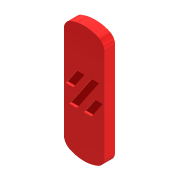
# Autodesk Inventor part: Cover_Squared
Saved by Autodesk Inventor 2021 (Build 250183000, 183)
## iProperties
Created: 2021-09-01
Part Number: Cover_Squared
Material: Generisch
Document SubType Name: Modeling
Designer: Rama
Density: 1 g/cm^3
Appearance: Hellrot
Author: Rama
Autodesk Inventor part; units mm, degrees
ref_plane "YZ Plane" through (0, 0, 0) normal (1, 0, 0) x (0, 1, 0)
ref_plane "XZ Plane" through (0, 0, 0) normal (0, 1, 0) x (-1, 0, 0)
ref_plane "XY Plane" through (0, 0, 0) normal (0, 0, 1) x (1, 0, 0)
sketch "Skizze1" plane through (0, 0, 0) normal (0, 0, 1) x (1, 0, 0)
  line L0 (7.75, -17.6806) -> (7.75, 17.6806) projected
  line L1 (-7.75, 17.6806) -> (-7.75, -17.6806) projected
  circle A0 centre (0, 0) radius 3.025 projected
  arc A1 (-5.3363, -21.3526) -> (5.3363, -21.3526) centre (0, -9) ccw projected
  arc A2 (5.3363, -21.3526) -> (7.75, -17.6806) centre (3.75, -17.6806) ccw projected
  arc A3 (7.75, 17.6806) -> (5.3363, 21.3526) centre (3.75, 17.6806) ccw projected
  arc A4 (5.3363, 21.3526) -> (-5.3363, 21.3526) centre (0, 9) ccw projected
  arc A5 (-5.3363, 21.3526) -> (-7.75, 17.6806) centre (-3.75, 17.6806) ccw projected
  arc A6 (-7.75, -17.6806) -> (-5.3363, -21.3526) centre (-3.75, -17.6806) ccw projected
  circle A7 centre (-0.25, 17) radius 1.7 projected
  circle A8 centre (-0.25, -7) radius 1.7 projected
  line L2 (5.34, 14.1) -> (3.3, 14.1) projected
  line L3 (3.3, 14.1) -> (3.3, 17.74) projected
  line L4 (3.3, 17.74) -> (5.34, 17.74) projected
  line L5 (5.34, 17.74) -> (5.34, 14.1) projected
  line L6 (-3.8, 14.1) -> (-5.84, 14.1) projected
  line L7 (-5.84, 14.1) -> (-5.84, 17.74) projected
  line L8 (-5.84, 17.74) -> (-3.8, 17.74) projected
  line L9 (-3.8, 17.74) -> (-3.8, 14.1) projected
  circle A9 centre (-0.25, -15.278) radius 2.9 projected
  point P0 (0, 0)
  point P1 (-17.1225, -5.975)
  point P2 (-17.1225, -12.025)
  point P3 (-17.1225, 6.3)
  point P4 (-17.1225, -14.3)
  point P5 (-17.1225, -17.7)
  constraints: 1 other
extrude "Extrusion1" add sketch "Skizze1" along normal blind 4 contours A2 A1 A6 L1 A5 A4 A3 L0 | A0 | A7 | A8 | L2 L3 L4 L5 | L6 L7 L8 L9 | A9
sketch "Skizze2" plane through (0, 0, 0) normal (0, 0, -1) x (-1, 0, 0)
  circle A0 centre (0, 0) radius 3.025 projected
  arc A1 (-5.3363, -21.3526) -> (5.3363, -21.3526) centre (0, -9) ccw projected
  arc A2 (-7.75, -17.6806) -> (-5.3363, -21.3526) centre (-3.75, -17.6806) ccw projected
  line L0 (-7.75, -17.6806) -> (-7.75, 17.6806) projected
  arc A3 (-5.3363, 21.3526) -> (-7.75, 17.6806) centre (-3.75, 17.6806) ccw projected
  arc A4 (5.3363, 21.3526) -> (-5.3363, 21.3526) centre (0, 9) ccw projected
  arc A5 (7.75, 17.6806) -> (5.3363, 21.3526) centre (3.75, 17.6806) ccw projected
  line L1 (7.75, 17.6806) -> (7.75, -17.6806) projected
  arc A6 (5.3363, -21.3526) -> (7.75, -17.6806) centre (3.75, -17.6806) ccw projected
  circle A7 centre (0.25, 17) radius 1.7 projected
  circle A8 centre (0.25, -7) radius 1.7 projected
  line L2 (-5.34, 14.1) -> (-3.3, 14.1) projected
  line L3 (-3.3, 14.1) -> (-3.3, 17.74) projected
  line L4 (-3.3, 17.74) -> (-5.34, 17.74) projected
  line L5 (-5.34, 17.74) -> (-5.34, 14.1) projected
  line L6 (3.8, 14.1) -> (5.84, 14.1) projected
  line L7 (5.84, 14.1) -> (5.84, 17.74) projected
  line L8 (5.84, 17.74) -> (3.8, 17.74) projected
  line L9 (3.8, 17.74) -> (3.8, 14.1) projected
  circle A9 centre (0.25, -15.278) radius 2.9 projected
  point P0 (0, 0)
extrude "Extrusion2" cut sketch "Skizze2" against normal blind 3.1 contours A0
sketch "Skizze3" plane through (0, 0, 0) normal (0, 0, -1) x (-1, 0, 0)
  circle A0 centre (0, 0) radius 3.025 projected
  arc A1 (-5.3363, -21.3526) -> (5.3363, -21.3526) centre (0, -9) ccw projected
  arc A2 (-7.75, -17.6806) -> (-5.3363, -21.3526) centre (-3.75, -17.6806) ccw projected
  line L0 (-7.75, -17.6806) -> (-7.75, 17.6806) projected
  arc A3 (-5.3363, 21.3526) -> (-7.75, 17.6806) centre (-3.75, 17.6806) ccw projected
  arc A4 (5.3363, 21.3526) -> (-5.3363, 21.3526) centre (0, 9) ccw projected
  arc A5 (7.75, 17.6806) -> (5.3363, 21.3526) centre (3.75, 17.6806) ccw projected
  line L1 (7.75, 17.6806) -> (7.75, -17.6806) projected
  arc A6 (5.3363, -21.3526) -> (7.75, -17.6806) centre (3.75, -17.6806) ccw projected
  circle A7 centre (0.25, 17) radius 1.7 projected
  circle A8 centre (0.25, -7) radius 1.7 projected
  line L2 (-5.34, 14.1) -> (-3.3, 14.1) projected
  line L3 (-3.3, 14.1) -> (-3.3, 17.74) projected
  line L4 (-3.3, 17.74) -> (-5.34, 17.74) projected
  line L5 (-5.34, 17.74) -> (-5.34, 14.1) projected
  line L6 (3.8, 14.1) -> (5.84, 14.1) projected
  line L7 (5.84, 14.1) -> (5.84, 17.74) projected
  line L8 (5.84, 17.74) -> (3.8, 17.74) projected
  line L9 (3.8, 17.74) -> (3.8, 14.1) projected
  circle A9 centre (0.25, -15.278) radius 2.9 projected
  point P0 (0, 0)
hole "Bohrung1" at (-0.25, 17, 0) at (-0.25, -7, 0) direction (0, 0, 1) diameter 5.6 depth 3.2 counterbore diameter 7.1 counterbore depth 1.2
sketch "Skizze4" plane through (0, 0, 4) normal (0, 0, 1) x (1, 0, 0)
  circle A0 centre (-0.25, 17) radius 3.55 projected
  circle A1 centre (-0.25, -7) radius 3.55 projected
  circle A2 centre (0, 0) radius 3.025 projected
  arc A3 (5.3363, -21.3526) -> (7.75, -17.6806) centre (3.75, -17.6806) ccw projected
  arc A4 (-5.3363, -21.3526) -> (5.3363, -21.3526) centre (0, -9) ccw projected
  arc A5 (-7.75, -17.6806) -> (-5.3363, -21.3526) centre (-3.75, -17.6806) ccw projected
  line L0 (-7.75, 17.6806) -> (-7.75, -17.6806) projected
  arc A6 (-5.3363, 21.3526) -> (-7.75, 17.6806) centre (-3.75, 17.6806) ccw projected
  arc A7 (5.3363, 21.3526) -> (-5.3363, 21.3526) centre (0, 9) ccw projected
  arc A8 (7.75, 17.6806) -> (5.3363, 21.3526) centre (3.75, 17.6806) ccw projected
  line L1 (7.75, -17.6806) -> (7.75, 17.6806) projected
  circle A9 centre (12.6079, -10) radius 2.8
  circle A10 centre (12.6079, -10) radius 2.8
  line L2 (4.1087, 0) -> (7.1087, 0)
  line L3 (7.1087, 0) -> (2.8877, -6.1994)
  line L4 (2.8877, -6.1994) -> (-0.1123, -6.1994)
  line L5 (-0.1123, -6.1994) -> (4.1087, 0)
  line L6 (2.721, 6.1994) -> (5.721, 6.1994)
  line L7 (5.721, 6.1994) -> (-2.721, -6.1994)
  line L8 (-2.721, -6.1994) -> (-5.721, -6.1994)
  line L9 (-5.721, -6.1994) -> (2.721, 6.1994)
  line L10 (-2.8877, 6.1994) -> (0.1123, 6.1994)
  line L11 (0.1123, 6.1994) -> (-4.1087, 0)
  line L12 (-4.1087, 0) -> (-7.1087, 0)
  line L13 (-7.1087, 0) -> (-2.8877, 6.1994)
  line L14 (7.1087, 6.1994) -> (7.1087, -6.1994)
  line L15 (7.1087, -6.1994) -> (-7.1087, -6.1994)
  line L16 (-7.1087, -6.1994) -> (-7.1087, 6.1994)
  line L17 (-7.1087, 6.1994) -> (7.1087, 6.1994)
  point P0 (0, 0)
  point P1 (16.5579, -10)
  point P2 (16.5579, -10)
  point P3 (16.5579, -10)
  point P4 (50.5428, -9.282)
  point P5 (-4.221, -6.1994)
  point P6 (4.221, 6.1994)
  point P7 (-1.3877, 6.1994)
  point P8 (1.3877, -6.1994)
  dimension "d89" = 5.6
  dimension "d104" = 5.6
  dimension "d107" = 14.2174
  dimension "d108" = 12.3988
  dimension "d109" = 2.1563
  dimension "d110" = 2.1563
  dimension "d111" = 2.4798
  dimension "d112" = 2.4798
  dimension "d113" = 2.4798
  dimension "d114" = 6.1994
  dimension "d115" = 6.1994
  dimension "d116" = 6.1994
  dimension "d117" = 15.5
  dimension "d118" = 0.6413
  constraints: 32 end point, 6 midpoint, 4 point on line, 2 centre point, 2 coincident, 2 parallel, 1 perpendicular
  measures "d89" diameter of A9
  measures "d104" diameter of A10
  measures "d107" distance between parallel lines of L14 L16
  measures "d108" distance between parallel lines of L15 L17
  measures "d109" distance between parallel lines of L7 L5
  measures "d110" distance between parallel lines of L11 L9
  measures "d111" distance between parallel lines of L9 L7
  measures "d112" distance between parallel lines of L5 L3
  measures "d113" distance between parallel lines of L13 L11
  measures "d114" distance between parallel lines of L15 L2
  measures "d115" distance between parallel lines of L17 L12
  measures "d116" distance from line of point (0, 0) L15
  measures "d117" distance between parallel lines of L1 L0
  measures "d118" distance between parallel lines of L0 L16
move faces "Verschieben1" translate (0, 0, 0.5) faces at (-2.5833, -5.8935, 4)
extrude "Extrusion4" cut sketch "Skizze4" along normal mid plane 0.8 contours L8 L9 A2 L7 A1 | A1 L7 L8 | L3 L4 L5 A1 | A1 L5 L2 L3 | A2 L9 L7 | A2 L9 L6 L7 | L13 L10 L11 L12
extrude "Extrusion5" cut sketch "Skizze4" along normal through all contours L8 L9 A2 L7 A1 | A1 L7 L8 | L3 L4 L5 A1 | A1 L5 L2 L3 | A2 L9 L7 | A2 L9 L6 L7 | L13 L10 L11 L12
sketch "Skizze5" plane through (0, 0, 0) normal (0, 0, -1) x (-1, 0, 0)
  circle A0 centre (0.25, -15.278) radius 2.9 projected
  point P0 (0, 0)
extrude "Extrusion6" cut sketch "Skizze5" against normal blind 1.4
chamfer "Fase2" distance 0.2 distance2 0.8 1 edges at (-0.25, -10.55, 0) measured on face at (6.175, 0, 0)
chamfer "Fase3" distance 2 distance2 0.4 1 edges at (-0.25, -9.8, 1.2) measured on face at (0.1992, -4.2363, 2.5333)
chamfer "Fase4" distance 2 distance2 0.4 1 edges at (-0.25, 14.2, 1.2) measured on face at (0.1992, 19.7637, 2.5333)
chamfer "Fase5" distance 0.2 distance2 0.8 1 edges at (-0.25, 13.45, 0) measured on face at (6.175, 0, 0)
chamfer "Fase6" distance 0.4 angle 45 8 edges at (-7.75, 0, 0) (-7.0925, -19.8777, 0) (0, -22.4559, 0) (7.0925, -19.8777, 0) (7.75, 0, 0) (7.0925, 19.8777, 0) (0, 22.4559, 0) (-7.0925, 19.8777, 0)
